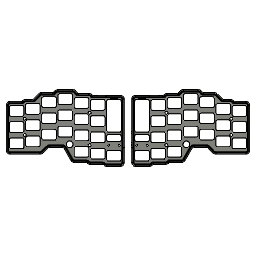
mriya-bumper-mjf-v1.17 (Autodesk Fusion 360 design; units mm, degrees)
Autodesk Fusion 360 part; units mm, degrees
(part 1 of 2)
sketch "mriya-bumper-mjf" plane through (0, 0, 0) normal (0, 0, 1) x (1, 0, 0)
  line L0 (-101.0213, 15.6719) -> (-94.7787, 21.9145) construction
  line L1 (-26.4858, 1.079) -> (-27.6142, 2.2074) construction
  line L2 (-138.1, 14.7932) -> (-103.1426, 14.7932) construction
  line L3 (-44.0716, 2.7932) -> (-29.0284, 2.7932) construction
  line L4 (-8.6, 0.4932) -> (-25.0716, 0.4932) construction
  line L5 (-64.4741, 6.1094) -> (-72.7517, 20.7608) construction
  line L6 (-45.4858, 3.379) -> (-46.6142, 4.5074) construction
  line L7 (-122.6142, 71.579) -> (-121.4858, 72.7074) construction
  line L8 (-101.0716, 81.2932) -> (-87.2284, 81.2932) construction
  line L9 (-138.1, 70.9932) -> (-124.0284, 70.9932) construction
  line L10 (-92.6574, 22.7932) -> (-76.2344, 22.7932) construction
  line L11 (-48.0284, 5.0932) -> (-62.7328, 5.0932) construction
  line L12 (-82.0716, 84.7932) -> (-64.7284, 84.7932) construction
  line L13 (-58.5716, 80.2932) -> (-45.7284, 80.2932) construction
  line L14 (-24.8, 19.4932) -> (-7.1, 19.4932) construction
  line L15 (-25.6, 20.2932) -> (-25.6, 77.9932) construction
  line L16 (-83.4858, 84.2074) -> (-85.8142, 81.879) construction
  line L17 (-63.3142, 84.2074) -> (-59.9858, 80.879) construction
  line L18 (-139.6, 69.4932) -> (-139.6, 16.2932) construction
  line L19 (-43.1858, 78.579) -> (-44.3142, 79.7074) construction
  line L20 (-99.4, 40.3932) -> (-99.4, 27.9932) construction
  line L21 (-98.6, 41.1932) -> (-86.2, 41.1932) construction
  line L22 (-98.6, 27.1932) -> (-86.2, 27.1932) construction
  line L23 (-85.4, 40.3932) -> (-85.4, 27.9932) construction
  line L24 (-42.4, 56.0932) -> (-42.4, 43.6932) construction
  line L25 (-41.6, 56.8932) -> (-29.2, 56.8932) construction
  line L26 (-41.6, 42.8932) -> (-29.2, 42.8932) construction
  line L27 (-28.4, 56.0932) -> (-28.4, 43.6932) construction
  line L28 (-61.4, 58.3932) -> (-61.4, 45.9932) construction
  line L29 (-60.6, 59.1932) -> (-48.2, 59.1932) construction
  line L30 (-60.6, 45.1932) -> (-48.2, 45.1932) construction
  line L31 (-47.4, 58.3932) -> (-47.4, 45.9932) construction
  line L32 (-137.4, 68.0932) -> (-137.4, 55.6932) construction
  line L33 (-136.6, 68.8932) -> (-124.2, 68.8932) construction
  line L34 (-136.6, 54.8932) -> (-124.2, 54.8932) construction
  line L35 (-123.4, 68.0932) -> (-123.4, 55.6932) construction
  line L36 (-61.4, 39.3932) -> (-61.4, 26.9932) construction
  line L37 (-60.6, 40.1932) -> (-48.2, 40.1932) construction
  line L38 (-60.6, 26.1932) -> (-48.2, 26.1932) construction
  line L39 (-47.4, 39.3932) -> (-47.4, 26.9932) construction
  line L40 (-42.4, 18.0932) -> (-42.4, 5.6932) construction
  line L41 (-41.6, 18.8932) -> (-29.2, 18.8932) construction
  line L42 (-41.6, 4.8932) -> (-29.2, 4.8932) construction
  line L43 (-28.4, 18.0932) -> (-28.4, 5.6932) construction
  line L44 (-23.4, 15.7932) -> (-23.4, 3.3932) construction
  line L45 (-22.6, 16.5932) -> (-10.2, 16.5932) construction
  line L46 (-22.6, 2.5932) -> (-10.2, 2.5932) construction
  line L47 (-9.4, 15.7932) -> (-9.4, 3.3932) construction
  line L48 (-137.4, 49.0932) -> (-137.4, 36.6932) construction
  line L49 (-136.6, 49.8932) -> (-124.2, 49.8932) construction
  line L50 (-136.6, 35.8932) -> (-124.2, 35.8932) construction
  line L51 (-123.4, 49.0932) -> (-123.4, 36.6932) construction
  line L52 (-118.4, 51.3932) -> (-118.4, 38.9932) construction
  line L53 (-117.6, 52.1932) -> (-105.2, 52.1932) construction
  line L54 (-117.6, 38.1932) -> (-105.2, 38.1932) construction
  line L55 (-104.4, 51.3932) -> (-104.4, 38.9932) construction
  line L56 (-137.4, 30.0932) -> (-137.4, 17.6932) construction
  line L57 (-136.6, 30.8932) -> (-124.2, 30.8932) construction
  line L58 (-136.6, 16.8932) -> (-124.2, 16.8932) construction
  line L59 (-123.4, 30.0932) -> (-123.4, 17.6932) construction
  line L60 (-61.4, 20.3932) -> (-61.4, 7.9932) construction
  line L61 (-60.6, 21.1932) -> (-48.2, 21.1932) construction
  line L62 (-60.6, 7.1932) -> (-48.2, 7.1932) construction
  line L63 (-47.4, 20.3932) -> (-47.4, 7.9932) construction
  line L64 (-80.4, 43.8932) -> (-80.4, 31.4932) construction
  line L65 (-79.6, 44.6932) -> (-67.2, 44.6932) construction
  line L66 (-79.6, 30.6932) -> (-67.2, 30.6932) construction
  line L67 (-66.4, 43.8932) -> (-66.4, 31.4932) construction
  line L68 (-80.4, 81.8932) -> (-80.4, 69.4932) construction
  line L69 (-79.6, 82.6932) -> (-67.2, 82.6932) construction
  line L70 (-79.6, 68.6932) -> (-67.2, 68.6932) construction
  line L71 (-66.4, 81.8932) -> (-66.4, 69.4932) construction
  line L72 (-42.4, 37.0932) -> (-42.4, 24.6932) construction
  line L73 (-41.6, 37.8932) -> (-29.2, 37.8932) construction
  line L74 (-41.6, 23.8932) -> (-29.2, 23.8932) construction
  line L75 (-28.4, 37.0932) -> (-28.4, 24.6932) construction
  line L76 (-118.4, 32.3932) -> (-118.4, 19.9932) construction
  line L77 (-117.6, 33.1932) -> (-105.2, 33.1932) construction
  line L78 (-117.6, 19.1932) -> (-105.2, 19.1932) construction
  line L79 (-104.4, 32.3932) -> (-104.4, 19.9932) construction
  line L80 (-61.4, 77.3932) -> (-61.4, 64.9932) construction
  line L81 (-60.6, 78.1932) -> (-48.2, 78.1932) construction
  line L82 (-60.6, 64.1932) -> (-48.2, 64.1932) construction
  line L83 (-47.4, 77.3932) -> (-47.4, 64.9932) construction
  line L84 (-42.4, 75.0932) -> (-42.4, 62.6932) construction
  line L85 (-41.6, 75.8932) -> (-29.2, 75.8932) construction
  line L86 (-41.6, 61.8932) -> (-29.2, 61.8932) construction
  line L87 (-28.4, 75.0932) -> (-28.4, 62.6932) construction
  line L88 (-118.4, 70.3932) -> (-118.4, 57.9932) construction
  line L89 (-117.6, 71.1932) -> (-105.2, 71.1932) construction
  line L90 (-117.6, 57.1932) -> (-105.2, 57.1932) construction
  line L91 (-104.4, 70.3932) -> (-104.4, 57.9932) construction
  line L92 (-99.4, 59.3932) -> (-99.4, 46.9932) construction
  line L93 (-98.6, 60.1932) -> (-86.2, 60.1932) construction
  line L94 (-98.6, 46.1932) -> (-86.2, 46.1932) construction
  line L95 (-85.4, 59.3932) -> (-85.4, 46.9932) construction
  line L96 (-80.4, 62.8932) -> (-80.4, 50.4932) construction
  line L97 (-79.6, 63.6932) -> (-67.2, 63.6932) construction
  line L98 (-79.6, 49.6932) -> (-67.2, 49.6932) construction
  line L99 (-66.4, 62.8932) -> (-66.4, 50.4932) construction
  line L100 (-99.4, 78.3932) -> (-99.4, 65.9932) construction
  line L101 (-98.6, 79.1932) -> (-86.2, 79.1932) construction
  line L102 (-98.6, 65.1932) -> (-86.2, 65.1932) construction
  line L103 (-85.4, 78.3932) -> (-85.4, 65.9932) construction
  circle A0 centre (-120.9, 53.5432) radius 1.7
  circle A1 centre (-120.9, 34.5432) radius 1.7
  circle A2 centre (-68.3, 23.4932) radius 3.9
  circle A3 centre (-44.9, 22.5432) radius 1.7
  circle A4 centre (-44.9, 60.5432) radius 1.7
  arc A5 (-43.1858, 78.579) -> (-41.7716, 77.9932) centre (-41.7716, 79.9932) ccw construction
  arc A6 (-44.3142, 79.7074) -> (-45.7284, 80.2932) centre (-45.7285, 78.2931) ccw construction
  arc A7 (-59.9858, 80.879) -> (-58.5716, 80.2932) centre (-58.5716, 82.2931) ccw construction
  arc A8 (-63.3142, 84.2074) -> (-64.7284, 84.7932) centre (-64.7285, 82.7931) ccw construction
  arc A9 (-82.0716, 84.7932) -> (-83.4858, 84.2074) centre (-82.0716, 82.7933) ccw construction
  arc A10 (-87.2284, 81.2932) -> (-85.8142, 81.879) centre (-87.2284, 83.2932) ccw construction
  arc A11 (-101.0716, 81.2932) -> (-102.4858, 80.7074) centre (-101.0716, 79.2933) ccw construction
  arc A12 (-120.0716, 73.2932) -> (-121.4858, 72.7074) centre (-120.0716, 71.2933) ccw construction
  arc A13 (-124.0284, 70.9932) -> (-122.6142, 71.579) centre (-124.0284, 72.9932) ccw construction
  arc A14 (-138.1, 70.9932) -> (-139.6, 69.4932) centre (-138.1, 69.4932) ccw construction
  arc A15 (-139.6, 16.2932) -> (-138.1, 14.7932) centre (-138.1, 16.2932) ccw construction
  arc A16 (-103.1426, 14.7932) -> (-101.0213, 15.6719) centre (-103.1426, 17.7931) ccw construction
  arc A17 (-92.6574, 22.7932) -> (-94.7787, 21.9145) centre (-92.6573, 19.7931) ccw construction
  arc A18 (-72.7517, 20.7608) -> (-76.2344, 22.7932) centre (-76.2344, 18.793) ccw construction
  arc A19 (-64.4741, 6.1094) -> (-62.7328, 5.0932) centre (-62.7328, 7.0932) ccw construction
  arc A20 (-46.6142, 4.5074) -> (-48.0284, 5.0932) centre (-48.0284, 3.0933) ccw construction
  arc A21 (-45.4858, 3.379) -> (-44.0716, 2.7932) centre (-44.0715, 4.7933) ccw construction
  arc A22 (-27.6142, 2.2074) -> (-29.0284, 2.7932) centre (-29.0284, 0.7933) ccw construction
  arc A23 (-26.4858, 1.079) -> (-25.0716, 0.4932) centre (-25.0715, 2.4933) ccw construction
  arc A24 (-8.6, 0.4932) -> (-7.1, 1.9932) centre (-8.6, 1.9932) ccw construction
  line L104 (-7.1, 1.9932) -> (-7.1, 76.4932) construction
  line L105 (-41.7716, 77.9932) -> (-8.6, 77.9932) construction
  arc A25 (-7.1, 76.4932) -> (-8.6, 77.9932) centre (-8.6, 76.4932) ccw construction
  arc A26 (-136.6, 68.8932) -> (-137.4, 68.0932) centre (-136.6, 68.0932) ccw construction
  arc A27 (-123.4, 68.0932) -> (-124.2, 68.8932) centre (-124.2, 68.0932) ccw construction
  arc A28 (-124.2, 54.8932) -> (-123.4, 55.6932) centre (-124.2, 55.6932) ccw construction
  arc A29 (-137.4, 55.6932) -> (-136.6, 54.8932) centre (-136.6, 55.6932) ccw construction
  arc A30 (-136.6, 49.8932) -> (-137.4, 49.0932) centre (-136.6, 49.0932) ccw construction
  arc A31 (-123.4, 49.0932) -> (-124.2, 49.8932) centre (-124.2, 49.0932) ccw construction
  arc A32 (-124.2, 35.8932) -> (-123.4, 36.6932) centre (-124.2, 36.6932) ccw construction
  arc A33 (-137.4, 36.6932) -> (-136.6, 35.8932) centre (-136.6, 36.6932) ccw construction
  arc A34 (-136.6, 30.8932) -> (-137.4, 30.0932) centre (-136.6, 30.0932) ccw construction
  arc A35 (-123.4, 30.0932) -> (-124.2, 30.8932) centre (-124.2, 30.0932) ccw construction
  arc A36 (-124.2, 16.8932) -> (-123.4, 17.6932) centre (-124.2, 17.6932) ccw construction
  arc A37 (-137.4, 17.6932) -> (-136.6, 16.8932) centre (-136.6, 17.6932) ccw construction
  arc A38 (-118.4, 19.9932) -> (-117.6, 19.1932) centre (-117.6, 19.9932) ccw construction
  arc A39 (-105.2, 19.1932) -> (-104.4, 19.9932) centre (-105.2, 19.9932) ccw construction
  arc A40 (-104.4, 32.3932) -> (-105.2, 33.1932) centre (-105.2, 32.3932) ccw construction
  arc A41 (-117.6, 33.1932) -> (-118.4, 32.3932) centre (-117.6, 32.3932) ccw construction
  arc A42 (-105.2, 38.1932) -> (-104.4, 38.9932) centre (-105.2, 38.9932) ccw construction
  arc A43 (-118.4, 38.9932) -> (-117.6, 38.1932) centre (-117.6, 38.9932) ccw construction
  arc A44 (-117.6, 52.1932) -> (-118.4, 51.3932) centre (-117.6, 51.3932) ccw construction
  arc A45 (-104.4, 51.3932) -> (-105.2, 52.1932) centre (-105.2, 51.3932) ccw construction
  arc A46 (-118.4, 57.9932) -> (-117.6, 57.1932) centre (-117.6, 57.9932) ccw construction
  arc A47 (-105.2, 57.1932) -> (-104.4, 57.9932) centre (-105.2, 57.9932) ccw construction
  arc A48 (-104.4, 70.3932) -> (-105.2, 71.1932) centre (-105.2, 70.3932) ccw construction
  arc A49 (-117.6, 71.1932) -> (-118.4, 70.3932) centre (-117.6, 70.3932) ccw construction
  arc A50 (-98.6, 79.1932) -> (-99.4, 78.3932) centre (-98.6, 78.3932) ccw construction
  arc A51 (-85.4, 78.3932) -> (-86.2, 79.1932) centre (-86.2, 78.3932) ccw construction
  arc A52 (-86.2, 65.1932) -> (-85.4, 65.9932) centre (-86.2, 65.9932) ccw construction
  arc A53 (-99.4, 65.9932) -> (-98.6, 65.1932) centre (-98.6, 65.9932) ccw construction
  arc A54 (-98.6, 60.1932) -> (-99.4, 59.3932) centre (-98.6, 59.3932) ccw construction
  arc A55 (-85.4, 59.3932) -> (-86.2, 60.1932) centre (-86.2, 59.3932) ccw construction
  arc A56 (-86.2, 46.1932) -> (-85.4, 46.9932) centre (-86.2, 46.9932) ccw construction
  arc A57 (-99.4, 46.9932) -> (-98.6, 46.1932) centre (-98.6, 46.9932) ccw construction
  arc A58 (-98.6, 41.1932) -> (-99.4, 40.3932) centre (-98.6, 40.3932) ccw construction
  arc A59 (-99.4, 27.9932) -> (-98.6, 27.1932) centre (-98.6, 27.9932) ccw construction
  arc A60 (-86.2, 27.1932) -> (-85.4, 27.9932) centre (-86.2, 27.9932) ccw construction
  arc A61 (-85.4, 40.3932) -> (-86.2, 41.1932) centre (-86.2, 40.3932) ccw construction
  arc A62 (-80.4, 31.4932) -> (-79.6, 30.6932) centre (-79.6, 31.4932) ccw construction
  arc A63 (-79.6, 44.6932) -> (-80.4, 43.8932) centre (-79.6, 43.8932) ccw construction
  arc A64 (-66.4, 43.8932) -> (-67.2, 44.6932) centre (-67.2, 43.8932) ccw construction
  arc A65 (-67.2, 30.6932) -> (-66.4, 31.4932) centre (-67.2, 31.4932) ccw construction
  arc A66 (-67.2, 49.6932) -> (-66.4, 50.4932) centre (-67.2, 50.4932) ccw construction
  arc A67 (-80.4, 50.4932) -> (-79.6, 49.6932) centre (-79.6, 50.4932) ccw construction
  arc A68 (-79.6, 63.6932) -> (-80.4, 62.8932) centre (-79.6, 62.8932) ccw construction
  arc A69 (-66.4, 62.8932) -> (-67.2, 63.6932) centre (-67.2, 62.8932) ccw construction
  arc A70 (-67.2, 68.6932) -> (-66.4, 69.4932) centre (-67.2, 69.4932) ccw construction
  arc A71 (-80.4, 69.4932) -> (-79.6, 68.6932) centre (-79.6, 69.4932) ccw construction
  arc A72 (-79.6, 82.6932) -> (-80.4, 81.8932) centre (-79.6, 81.8932) ccw construction
  arc A73 (-66.4, 81.8932) -> (-67.2, 82.6932) centre (-67.2, 81.8932) ccw construction
  arc A74 (-60.6, 78.1932) -> (-61.4, 77.3932) centre (-60.6, 77.3932) ccw construction
  arc A75 (-61.4, 64.9932) -> (-60.6, 64.1932) centre (-60.6, 64.9932) ccw construction
  arc A76 (-48.2, 64.1932) -> (-47.4, 64.9932) centre (-48.2, 64.9932) ccw construction
  arc A77 (-47.4, 77.3932) -> (-48.2, 78.1932) centre (-48.2, 77.3932) ccw construction
  arc A78 (-47.4, 58.3932) -> (-48.2, 59.1932) centre (-48.2, 58.3932) ccw construction
  arc A79 (-60.6, 59.1932) -> (-61.4, 58.3932) centre (-60.6, 58.3932) ccw construction
  arc A80 (-61.4, 45.9932) -> (-60.6, 45.1932) centre (-60.6, 45.9932) ccw construction
  arc A81 (-48.2, 45.1932) -> (-47.4, 45.9932) centre (-48.2, 45.9932) ccw construction
  arc A82 (-47.4, 39.3932) -> (-48.2, 40.1932) centre (-48.2, 39.3932) ccw construction
  arc A83 (-60.6, 40.1932) -> (-61.4, 39.3932) centre (-60.6, 39.3932) ccw construction
  arc A84 (-61.4, 26.9932) -> (-60.6, 26.1932) centre (-60.6, 26.9932) ccw construction
  arc A85 (-48.2, 26.1932) -> (-47.4, 26.9932) centre (-48.2, 26.9932) ccw construction
  arc A86 (-47.4, 20.3932) -> (-48.2, 21.1932) centre (-48.2, 20.3932) ccw construction
  arc A87 (-60.6, 21.1932) -> (-61.4, 20.3932) centre (-60.6, 20.3932) ccw construction
  arc A88 (-61.4, 7.9932) -> (-60.6, 7.1932) centre (-60.6, 7.9932) ccw construction
  arc A89 (-48.2, 7.1932) -> (-47.4, 7.9932) centre (-48.2, 7.9932) ccw construction
  arc A90 (-42.4, 5.6932) -> (-41.6, 4.8932) centre (-41.6, 5.6932) ccw construction
  arc A91 (-29.2, 4.8932) -> (-28.4, 5.6932) centre (-29.2, 5.6932) ccw construction
  arc A92 (-28.4, 18.0932) -> (-29.2, 18.8932) centre (-29.2, 18.0932) ccw construction
  arc A93 (-41.6, 18.8932) -> (-42.4, 18.0932) centre (-41.6, 18.0932) ccw construction
  arc A94 (-23.4, 3.3932) -> (-22.6, 2.5932) centre (-22.6, 3.3932) ccw construction
  arc A95 (-10.2, 2.5932) -> (-9.4, 3.3932) centre (-10.2, 3.3932) ccw construction
  arc A96 (-9.4, 15.7932) -> (-10.2, 16.5932) centre (-10.2, 15.7932) ccw construction
  arc A97 (-22.6, 16.5932) -> (-23.4, 15.7932) centre (-22.6, 15.7932) ccw construction
  arc A98 (-29.2, 23.8932) -> (-28.4, 24.6932) centre (-29.2, 24.6932) ccw construction
  arc A99 (-42.4, 24.6932) -> (-41.6, 23.8932) centre (-41.6, 24.6932) ccw construction
  arc A100 (-41.6, 37.8932) -> (-42.4, 37.0932) centre (-41.6, 37.0932) ccw construction
  arc A101 (-28.4, 37.0932) -> (-29.2, 37.8932) centre (-29.2, 37.0932) ccw construction
  arc A102 (-29.2, 42.8932) -> (-28.4, 43.6932) centre (-29.2, 43.6932) ccw construction
  arc A103 (-42.4, 43.6932) -> (-41.6, 42.8932) centre (-41.6, 43.6932) ccw construction
  arc A104 (-41.6, 56.8932) -> (-42.4, 56.0932) centre (-41.6, 56.0932) ccw construction
  arc A105 (-28.4, 56.0932) -> (-29.2, 56.8932) centre (-29.2, 56.0932) ccw construction
  arc A106 (-29.2, 61.8932) -> (-28.4, 62.6932) centre (-29.2, 62.6932) ccw construction
  arc A107 (-42.4, 62.6932) -> (-41.6, 61.8932) centre (-41.6, 62.6932) ccw construction
  arc A108 (-41.6, 75.8932) -> (-42.4, 75.0932) centre (-41.6, 75.0932) ccw construction
  arc A109 (-28.4, 75.0932) -> (-29.2, 75.8932) centre (-29.2, 75.0932) ccw construction
  circle A110 centre (-22.6, 22.4932) radius 1.1
  circle A111 centre (-10.1, 22.4932) radius 1.1
  line L106 (-102.4858, 80.7074) -> (-109.0213, 74.1719) construction
  line L107 (-120.0716, 73.2932) -> (-111.1426, 73.2932) construction
  arc A112 (-111.1426, 73.2932) -> (-109.0213, 74.1719) centre (-111.1426, 76.2932) ccw construction
  arc A113 (-64.7284, 82.7932) -> (-64.7285, 82.7932) centre (-64.7285, 82.7931) ccw
  arc A114 (-45.7284, 78.2932) -> (-45.7285, 78.2932) centre (-45.7285, 78.2931) ccw
  arc A115 (-25.0716, 2.4932) -> (-25.0715, 2.4932) centre (-25.0715, 2.4933) ccw
  arc A116 (-44.0716, 4.7932) -> (-44.0715, 4.7932) centre (-44.0715, 4.7933) ccw
  line L108 (-138.9, 58.3932) -> (-138.9, 66.8932)
  line L109 (-136.9, 68.8932) -> (-123.9, 68.8932)
  arc A117 (-121.9, 66.8932) -> (-123.9, 68.8932) centre (-123.9, 66.8932) ccw
  arc A118 (-136.9, 68.8932) -> (-138.9, 66.8932) centre (-136.9, 66.8932) ccw
  line L110 (-104.9, 58.6932) -> (-117.9, 58.6932)
  line L111 (-119.9, 60.6932) -> (-119.9, 69.1932)
  arc A119 (-117.9, 71.1932) -> (-119.9, 69.1932) centre (-117.9, 69.1932) ccw
  line L112 (-117.9, 71.1932) -> (-104.9, 71.1932)
  arc A120 (-102.9, 69.1932) -> (-104.9, 71.1932) centre (-104.9, 69.1932) ccw
  line L113 (-102.9, 69.1932) -> (-102.9, 60.6932)
  line L114 (-85.9, 66.6932) -> (-98.9, 66.6932)
  line L115 (-100.9, 68.6932) -> (-100.9, 77.1932)
  arc A121 (-98.9, 79.1932) -> (-100.9, 77.1932) centre (-98.9, 77.1932) ccw
  line L116 (-98.9, 79.1932) -> (-85.9, 79.1932)
  arc A122 (-83.9, 77.1932) -> (-85.9, 79.1932) centre (-85.9, 77.1932) ccw
  line L117 (-83.9, 77.1932) -> (-83.9, 68.6932)
  line L118 (-66.9, 70.1932) -> (-79.9, 70.1932)
  line L119 (-81.9, 72.1932) -> (-81.9, 80.6932)
  arc A123 (-79.9, 82.6932) -> (-81.9, 80.6932) centre (-79.9, 80.6932) ccw
  line L120 (-79.9, 82.6932) -> (-66.9, 82.6932)
  arc A124 (-64.9, 80.6932) -> (-66.9, 82.6932) centre (-66.9, 80.6932) ccw
  line L121 (-64.9, 80.6932) -> (-64.9, 72.1932)
  line L122 (-47.9, 65.6932) -> (-60.9, 65.6932)
  line L123 (-62.9, 67.6932) -> (-62.9, 76.1932)
  arc A125 (-60.9, 78.1932) -> (-62.9, 76.1932) centre (-60.9, 76.1932) ccw
  line L124 (-60.9, 78.1932) -> (-47.9, 78.1932)
  arc A126 (-45.9, 76.1932) -> (-47.9, 78.1932) centre (-47.9, 76.1932) ccw
  line L125 (-45.9, 76.1932) -> (-45.9, 67.6932)
  line L126 (-43.9, 65.3932) -> (-43.9, 73.8932)
  arc A127 (-41.9, 75.8932) -> (-43.9, 73.8932) centre (-41.9, 73.8932) ccw
  line L127 (-41.9, 75.8932) -> (-28.9, 75.8932)
  arc A128 (-26.9, 73.8932) -> (-28.9, 75.8932) centre (-28.9, 73.8932) ccw
  line L128 (-26.9, 73.8932) -> (-26.9, 65.3932)
  arc A129 (-9.9, 26.8932) -> (-7.9, 28.8932) centre (-9.9, 28.8932) ccw
  line L129 (-9.9, 26.8932) -> (-22.9, 26.8932)
  arc A130 (-24.9, 28.8932) -> (-22.9, 26.8932) centre (-22.9, 28.8932) ccw
  arc A131 (-22.9, 75.8932) -> (-24.9, 73.8932) centre (-22.9, 73.8932) ccw
  arc A132 (-7.9, 73.8932) -> (-9.9, 75.8932) centre (-9.9, 73.8932) ccw
  line L130 (-28.9, 63.3932) -> (-41.9, 63.3932)
  line L131 (-121.9, 66.8932) -> (-121.9, 58.3932)
  line L132 (-123.9, 56.3932) -> (-136.9, 56.3932)
  line L133 (-122.6849, 71.6497) -> (-121.5565, 72.7781)
  arc A133 (-120.0716, 73.3932) -> (-121.5565, 72.7781) centre (-120.0716, 71.2933) ccw
  line L134 (-120.0716, 73.3932) -> (-111.1426, 73.3932)
  arc A134 (-111.1426, 73.3932) -> (-109.092, 74.2426) centre (-111.1426, 76.2932) ccw
  line L135 (-102.5565, 80.7781) -> (-109.092, 74.2426)
  arc A135 (-101.0716, 81.3932) -> (-102.5565, 80.7781) centre (-101.0716, 79.2933) ccw
  line L136 (-101.0716, 81.3932) -> (-87.2284, 81.3932)
  arc A136 (-87.2284, 81.3932) -> (-85.8849, 81.9497) centre (-87.2284, 83.2932) ccw
  line L137 (-83.5565, 84.2781) -> (-85.8849, 81.9497)
  arc A137 (-82.0716, 84.8932) -> (-83.5565, 84.2781) centre (-82.0716, 82.7933) ccw
  line L138 (-82.0716, 84.8932) -> (-64.7284, 84.8932)
  arc A138 (-63.2435, 84.2781) -> (-64.7284, 84.8932) centre (-64.7285, 82.7931) ccw
  line L139 (-63.2435, 84.2781) -> (-59.9151, 80.9497)
  arc A139 (-59.9151, 80.9497) -> (-58.5716, 80.3932) centre (-58.5716, 82.2931) ccw
  line L140 (-58.5716, 80.3932) -> (-45.7284, 80.3932)
  arc A140 (-44.2435, 79.7781) -> (-45.7284, 80.3932) centre (-45.7285, 78.2931) ccw
  line L141 (-43.1151, 78.6497) -> (-44.2435, 79.7781)
  arc A141 (-43.1151, 78.6497) -> (-41.7716, 78.0932) centre (-41.7716, 79.9932) ccw
  line L142 (-41.7716, 78.0932) -> (-8.6, 78.0932)
  arc A142 (-7, 76.4932) -> (-8.6, 78.0932) centre (-8.6, 76.4932) ccw
  line L143 (-7, 1.9932) -> (-7, 76.4932)
  arc A143 (-8.6, 0.3932) -> (-7, 1.9932) centre (-8.6, 1.9932) ccw
  line L144 (-8.6, 0.3932) -> (-25.0716, 0.3932)
  arc A144 (-26.5565, 1.0083) -> (-25.0716, 0.3932) centre (-25.0715, 2.4933) ccw
  line L145 (-26.5565, 1.0083) -> (-27.6849, 2.1367)
  arc A145 (-27.6849, 2.1367) -> (-29.0284, 2.6932) centre (-29.0284, 0.7933) ccw
  line L146 (-44.0716, 2.6932) -> (-29.0284, 2.6932)
  arc A146 (-45.5565, 3.3083) -> (-44.0716, 2.6932) centre (-44.0715, 4.7933) ccw
  line L147 (-45.5565, 3.3083) -> (-46.6849, 4.4367)
  arc A147 (-46.6849, 4.4367) -> (-48.0284, 4.9932) centre (-48.0284, 3.0933) ccw
  line L148 (-48.0284, 4.9932) -> (-62.7328, 4.9932)
  arc A148 (-64.5612, 6.0602) -> (-62.7328, 4.9932) centre (-62.7328, 7.0932) ccw
  line L149 (-64.5612, 6.0602) -> (-72.8388, 20.7116)
  arc A149 (-72.8388, 20.7116) -> (-76.2344, 22.6932) centre (-76.2344, 18.793) ccw
  line L150 (-92.6574, 22.6932) -> (-76.2344, 22.6932)
  arc A150 (-92.6574, 22.6932) -> (-94.708, 21.8438) centre (-92.6573, 19.7931) ccw
  line L151 (-100.9506, 15.6012) -> (-94.708, 21.8438)
  arc A151 (-103.1426, 14.6932) -> (-100.9506, 15.6012) centre (-103.1426, 17.7931) ccw
  line L152 (-138.1, 14.6932) -> (-103.1426, 14.6932)
  arc A152 (-139.7, 16.2932) -> (-138.1, 14.6932) centre (-138.1, 16.2932) ccw
  line L153 (-139.7, 69.4932) -> (-139.7, 16.2932)
  arc A153 (-138.1, 71.0932) -> (-139.7, 69.4932) centre (-138.1, 69.4932) ccw
  line L154 (-138.1, 71.0932) -> (-124.0284, 71.0932)
  arc A154 (-124.0284, 71.0932) -> (-122.6849, 71.6497) centre (-124.0284, 72.9932) ccw
  line L155 (-22.9, 34.8932) -> (-9.9, 34.8932)
  line L156 (-24.9, 28.8932) -> (-24.9, 32.8932)
  line L157 (-24.9, 39.8932) -> (-24.9, 73.8932)
  line L158 (-7.9, 73.8932) -> (-7.9, 39.8932)
  line L159 (-7.9, 32.8932) -> (-7.9, 28.8932)
  arc A155 (-24.9, 39.8932) -> (-22.9, 37.8932) centre (-22.9, 39.8932) ccw
  arc A156 (-9.9, 37.8932) -> (-7.9, 39.8932) centre (-9.9, 39.8932) ccw
  arc A157 (-22.9, 34.8932) -> (-24.9, 32.8932) centre (-22.9, 32.8932) ccw
  arc A158 (-7.9, 32.8932) -> (-9.9, 34.8932) centre (-9.9, 32.8932) ccw
  circle A159 centre (-22.6, 22.4932) radius 2.1
  circle A160 centre (-10.1, 22.4932) radius 2.1
  arc A161 (-25.6, 20.2932) -> (-24.8, 19.4932) centre (-24.8, 20.2932) ccw construction
  arc A162 (-138.9, 58.3932) -> (-136.9, 56.3932) centre (-136.9, 58.3932) ccw
  arc A163 (-123.9, 56.3932) -> (-121.9, 58.3932) centre (-123.9, 58.3932) ccw
  arc A164 (-119.9, 60.6932) -> (-117.9, 58.6932) centre (-117.9, 60.6932) ccw
  arc A165 (-104.9, 58.6932) -> (-102.9, 60.6932) centre (-104.9, 60.6932) ccw
  arc A166 (-100.9, 68.6932) -> (-98.9, 66.6932) centre (-98.9, 68.6932) ccw
  arc A167 (-85.9, 66.6932) -> (-83.9, 68.6932) centre (-85.9, 68.6932) ccw
  arc A168 (-81.9, 72.1932) -> (-79.9, 70.1932) centre (-79.9, 72.1932) ccw
  arc A169 (-66.9, 70.1932) -> (-64.9, 72.1932) centre (-66.9, 72.1932) ccw
  arc A170 (-62.9, 67.6932) -> (-60.9, 65.6932) centre (-60.9, 67.6932) ccw
  arc A171 (-47.9, 65.6932) -> (-45.9, 67.6932) centre (-47.9, 67.6932) ccw
  arc A172 (-43.9, 65.3932) -> (-41.9, 63.3932) centre (-41.9, 65.3932) ccw
  arc A173 (-28.9, 63.3932) -> (-26.9, 65.3932) centre (-28.9, 65.3932) ccw
  line L160 (-121.9, 47.8932) -> (-121.9, 39.3932)
  arc A174 (-121.9, 47.8932) -> (-123.9, 49.8932) centre (-123.9, 47.8932) ccw
  line L161 (-136.9, 49.8932) -> (-123.9, 49.8932)
  arc A175 (-136.9, 49.8932) -> (-138.9, 47.8932) centre (-136.9, 47.8932) ccw
  line L162 (-138.9, 39.3932) -> (-138.9, 47.8932)
  arc A176 (-138.9, 39.3932) -> (-136.9, 37.3932) centre (-136.9, 39.3932) ccw
  line L163 (-123.9, 37.3932) -> (-136.9, 37.3932)
  arc A177 (-123.9, 37.3932) -> (-121.9, 39.3932) centre (-123.9, 39.3932) ccw
  arc A178 (-104.9, 39.6932) -> (-102.9, 41.6932) centre (-104.9, 41.6932) ccw
  line L164 (-104.9, 39.6932) -> (-117.9, 39.6932)
  arc A179 (-119.9, 41.6932) -> (-117.9, 39.6932) centre (-117.9, 41.6932) ccw
  line L165 (-119.9, 41.6932) -> (-119.9, 49.7719)
  line L166 (-117.4787, 52.1932) -> (-104.9, 52.1932)
  arc A180 (-102.9, 50.1932) -> (-104.9, 52.1932) centre (-104.9, 50.1932) ccw
  line L167 (-102.9, 50.1932) -> (-102.9, 41.6932)
  arc A181 (-85.9, 47.6932) -> (-83.9, 49.6932) centre (-85.9, 49.6932) ccw
  line L168 (-85.9, 47.6932) -> (-98.9, 47.6932)
  arc A182 (-100.9, 49.6932) -> (-98.9, 47.6932) centre (-98.9, 49.6932) ccw
  line L169 (-100.9, 49.6932) -> (-100.9, 58.1932)
  arc A183 (-98.9, 60.1932) -> (-100.9, 58.1932) centre (-98.9, 58.1932) ccw
  line L170 (-98.9, 60.1932) -> (-85.9, 60.1932)
  arc A184 (-83.9, 58.1932) -> (-85.9, 60.1932) centre (-85.9, 58.1932) ccw
  line L171 (-83.9, 58.1932) -> (-83.9, 49.6932)
  arc A185 (-79.9, 63.6932) -> (-81.9, 61.6932) centre (-79.9, 61.6932) ccw
  line L172 (-79.9, 63.6932) -> (-66.9, 63.6932)
  arc A186 (-64.9, 61.6932) -> (-66.9, 63.6932) centre (-66.9, 61.6932) ccw
  line L173 (-64.9, 61.6932) -> (-64.9, 53.1932)
  arc A187 (-66.9, 51.1932) -> (-64.9, 53.1932) centre (-66.9, 53.1932) ccw
  line L174 (-66.9, 51.1932) -> (-79.9, 51.1932)
  arc A188 (-81.9, 53.1932) -> (-79.9, 51.1932) centre (-79.9, 53.1932) ccw
  line L175 (-81.9, 53.1932) -> (-81.9, 61.6932)
  arc A189 (-60.9, 59.1932) -> (-62.9, 57.1932) centre (-60.9, 57.1932) ccw
  line L176 (-60.9, 59.1932) -> (-48.3213, 59.1932)
  line L177 (-45.9, 56.7719) -> (-45.9, 48.6932)
  arc A190 (-47.9, 46.6932) -> (-45.9, 48.6932) centre (-47.9, 48.6932) ccw
  line L178 (-47.9, 46.6932) -> (-60.9, 46.6932)
  arc A191 (-62.9, 48.6932) -> (-60.9, 46.6932) centre (-60.9, 48.6932) ccw
  line L179 (-62.9, 48.6932) -> (-62.9, 57.1932)
  arc A192 (-41.9, 56.8932) -> (-43.9, 54.8932) centre (-41.9, 54.8932) ccw
  line L180 (-41.9, 56.8932) -> (-28.9, 56.8932)
  arc A193 (-26.9, 54.8932) -> (-28.9, 56.8932) centre (-28.9, 54.8932) ccw
  line L181 (-26.9, 54.8932) -> (-26.9, 46.3932)
  arc A194 (-28.9, 44.3932) -> (-26.9, 46.3932) centre (-28.9, 46.3932) ccw
  line L182 (-28.9, 44.3932) -> (-41.9, 44.3932)
  arc A195 (-43.9, 46.3932) -> (-41.9, 44.3932) centre (-41.9, 46.3932) ccw
  line L183 (-43.9, 46.3932) -> (-43.9, 54.8932)
  arc A196 (-123.9, 18.3932) -> (-121.9, 20.3932) centre (-123.9, 20.3932) ccw
  line L184 (-123.9, 18.3932) -> (-136.9, 18.3932)
  arc A197 (-138.9, 20.3932) -> (-136.9, 18.3932) centre (-136.9, 20.3932) ccw
  line L185 (-138.9, 20.3932) -> (-138.9, 28.8932)
  arc A198 (-136.9, 30.8932) -> (-138.9, 28.8932) centre (-136.9, 28.8932) ccw
  line L186 (-136.9, 30.8932) -> (-123.9, 30.8932)
  arc A199 (-121.9, 28.8932) -> (-123.9, 30.8932) centre (-123.9, 28.8932) ccw
  line L187 (-121.9, 28.8932) -> (-121.9, 20.3932)
  arc A200 (-104.9, 20.6932) -> (-102.9, 22.6932) centre (-104.9, 22.6932) ccw
  line L188 (-104.9, 20.6932) -> (-117.9, 20.6932)
  arc A201 (-119.9, 22.6932) -> (-117.9, 20.6932) centre (-117.9, 22.6932) ccw
  line L189 (-119.9, 22.6932) -> (-119.9, 30.7719)
  line L190 (-117.4787, 33.1932) -> (-104.9, 33.1932)
  arc A202 (-102.9, 31.1932) -> (-104.9, 33.1932) centre (-104.9, 31.1932) ccw
  line L191 (-102.9, 31.1932) -> (-102.9, 22.6932)
  arc A203 (-85.9, 28.6932) -> (-83.9, 30.6932) centre (-85.9, 30.6932) ccw
  line L192 (-85.9, 28.6932) -> (-98.9, 28.6932)
  arc A204 (-100.9, 30.6932) -> (-98.9, 28.6932) centre (-98.9, 30.6932) ccw
  line L193 (-100.9, 30.6932) -> (-100.9, 39.1932)
  arc A205 (-98.9, 41.1932) -> (-100.9, 39.1932) centre (-98.9, 39.1932) ccw
  line L194 (-98.9, 41.1932) -> (-85.9, 41.1932)
  arc A206 (-83.9, 39.1932) -> (-85.9, 41.1932) centre (-85.9, 39.1932) ccw
  line L195 (-83.9, 39.1932) -> (-83.9, 30.6932)
  arc A207 (-66.9, 32.1932) -> (-64.9, 34.1932) centre (-66.9, 34.1932) ccw
  line L196 (-66.9, 32.1932) -> (-79.9, 32.1932)
  arc A208 (-81.9, 34.1932) -> (-79.9, 32.1932) centre (-79.9, 34.1932) ccw
  line L197 (-81.9, 34.1932) -> (-81.9, 42.6932)
  arc A209 (-79.9, 44.6932) -> (-81.9, 42.6932) centre (-79.9, 42.6932) ccw
  line L198 (-79.9, 44.6932) -> (-66.9, 44.6932)
  arc A210 (-64.9, 42.6932) -> (-66.9, 44.6932) centre (-66.9, 42.6932) ccw
  line L199 (-64.9, 42.6932) -> (-64.9, 34.1932)
  arc A211 (-47.9, 27.6932) -> (-45.9, 29.6932) centre (-47.9, 29.6932) ccw
  line L200 (-47.9, 27.6932) -> (-60.9, 27.6932)
  arc A212 (-62.9, 29.6932) -> (-60.9, 27.6932) centre (-60.9, 29.6932) ccw
  line L201 (-62.9, 29.6932) -> (-62.9, 38.1932)
  arc A213 (-60.9, 40.1932) -> (-62.9, 38.1932) centre (-60.9, 38.1932) ccw
  line L202 (-60.9, 40.1932) -> (-47.9, 40.1932)
  arc A214 (-45.9, 38.1932) -> (-47.9, 40.1932) centre (-47.9, 38.1932) ccw
  line L203 (-45.9, 38.1932) -> (-45.9, 29.6932)
  arc A215 (-28.9, 25.3932) -> (-26.9, 27.3932) centre (-28.9, 27.3932) ccw
  line L204 (-28.9, 25.3932) -> (-41.9, 25.3932)
  arc A216 (-43.9, 27.3932) -> (-41.9, 25.3932) centre (-41.9, 27.3932) ccw
  line L205 (-43.9, 27.3932) -> (-43.9, 35.8932)
  arc A217 (-41.9, 37.8932) -> (-43.9, 35.8932) centre (-41.9, 35.8932) ccw
  line L206 (-41.9, 37.8932) -> (-28.9, 37.8932)
  arc A218 (-26.9, 35.8932) -> (-28.9, 37.8932) centre (-28.9, 35.8932) ccw
  line L207 (-26.9, 35.8932) -> (-26.9, 27.3932)
  arc A219 (-60.9, 21.1932) -> (-62.9, 19.1932) centre (-60.9, 19.1932) ccw
  line L208 (-62.9, 10.6932) -> (-62.9, 19.1932)
  arc A220 (-62.9, 10.6932) -> (-60.9, 8.6932) centre (-60.9, 10.6932) ccw
  line L209 (-47.9, 8.6932) -> (-60.9, 8.6932)
  arc A221 (-47.9, 8.6932) -> (-45.9, 10.6932) centre (-47.9, 10.6932) ccw
  line L210 (-28.9, 6.3932) -> (-41.9, 6.3932)
  arc A222 (-28.9, 6.3932) -> (-26.9, 8.3932) centre (-28.9, 8.3932) ccw
  line L211 (-26.9, 16.8932) -> (-26.9, 8.3932)
  arc A223 (-26.9, 16.8932) -> (-28.9, 18.8932) centre (-28.9, 16.8932) ccw
  line L212 (-41.9, 18.8932) -> (-28.9, 18.8932)
  arc A224 (-41.9, 18.8932) -> (-43.9, 16.8932) centre (-41.9, 16.8932) ccw
  line L213 (-43.9, 8.3932) -> (-43.9, 16.8932)
  arc A225 (-43.9, 8.3932) -> (-41.9, 6.3932) centre (-41.9, 8.3932) ccw
  arc A226 (-9.9, 4.0932) -> (-7.9, 6.0932) centre (-9.9, 6.0932) ccw
  line L214 (-9.9, 4.0932) -> (-22.9, 4.0932)
  arc A227 (-24.9, 6.0932) -> (-22.9, 4.0932) centre (-22.9, 6.0932) ccw
  line L215 (-24.9, 6.0932) -> (-24.9, 14.5932)
  arc A228 (-22.9, 16.5932) -> (-24.9, 14.5932) centre (-22.9, 14.5932) ccw
  line L216 (-22.9, 16.5932) -> (-9.9, 16.5932)
  arc A229 (-7.9, 14.5932) -> (-9.9, 16.5932) centre (-9.9, 14.5932) ccw
  line L217 (-7.9, 14.5932) -> (-7.9, 6.0932)
  line L218 (-60.9, 21.1932) -> (-48.3213, 21.1932)
  line L219 (-45.9, 18.7719) -> (-45.9, 10.6932)
  line L220 (-47.2607, 20.7539) -> (-46.3393, 19.8325)
  arc A230 (-47.2607, 20.7539) -> (-48.3213, 21.1932) centre (-48.3213, 19.6932) ccw
  arc A231 (-45.9, 18.7719) -> (-46.3393, 19.8325) centre (-47.4, 18.7719) ccw
  line L221 (-47.2607, 58.7539) -> (-46.3393, 57.8325)
  arc A232 (-47.2607, 58.7539) -> (-48.3213, 59.1932) centre (-48.3213, 57.6932) ccw
  arc A233 (-45.9, 56.7719) -> (-46.3393, 57.8325) centre (-47.4, 56.7719) ccw
  line L222 (-119.4607, 31.8325) -> (-118.5393, 32.7539)
  arc A234 (-119.4607, 31.8325) -> (-119.9, 30.7719) centre (-118.4, 30.7719) ccw
  arc A235 (-117.4787, 33.1932) -> (-118.5393, 32.7539) centre (-117.4787, 31.6932) ccw
  line L223 (-119.4607, 50.8325) -> (-118.5393, 51.7539)
  arc A236 (-117.4787, 52.1932) -> (-118.5393, 51.7539) centre (-117.4787, 50.6932) ccw
  arc A237 (-119.4607, 50.8325) -> (-119.9, 49.7719) centre (-118.4, 49.7719) ccw
  line L224 (-22.9, 75.8932) -> (-9.9, 75.8932)
  line L225 (-22.9, 37.8932) -> (-9.9, 37.8932)
  arc A238 (-101.0716, 83.9932) -> (-104.395, 82.6166) centre (-101.0716, 79.2933) ccw
  line L226 (-101.0716, 83.9932) -> (-88.1397, 83.9932)
  line L227 (-85.395, 86.1166) -> (-87.079, 84.4325)
  arc A239 (-82.0716, 87.4932) -> (-85.395, 86.1166) centre (-82.0716, 82.7933) ccw
  line L228 (-82.0716, 87.4932) -> (-64.7284, 87.4932)
  arc A240 (-61.405, 86.1166) -> (-64.7284, 87.4932) centre (-64.7285, 82.7931) ccw
  line L229 (-61.405, 86.1166) -> (-58.721, 83.4325)
  line L230 (-57.6603, 82.9932) -> (-45.7284, 82.9932)
  arc A241 (-42.405, 81.6166) -> (-45.7284, 82.9932) centre (-45.7285, 78.2931) ccw
  line L231 (-41.921, 81.1325) -> (-42.405, 81.6166)
  line L232 (-40.8603, 80.6932) -> (-8.6, 80.6932)
  arc A242 (-4.4, 76.4932) -> (-8.6, 80.6932) centre (-8.6, 76.4932) ccw
  line L233 (-4.4, 1.9932) -> (-4.4, 76.4932)
  arc A243 (-8.6, -2.2068) -> (-4.4, 1.9932) centre (-8.6, 1.9932) ccw
  line L234 (-8.6, -2.2068) -> (-25.0716, -2.2068)
  arc A244 (-28.395, -0.8302) -> (-25.0716, -2.2068) centre (-25.0715, 2.4933) ccw
  line L235 (-28.395, -0.8302) -> (-28.879, -0.3461)
  line L236 (-44.0716, 0.0932) -> (-29.9397, 0.0932)
  arc A245 (-47.395, 1.4698) -> (-44.0716, 0.0932) centre (-44.0715, 4.7933) ccw
  line L237 (-47.395, 1.4698) -> (-47.879, 1.9539)
  line L238 (-48.9397, 2.3932) -> (-62.7328, 2.3932)
  arc A246 (-66.8249, 4.7813) -> (-62.7328, 2.3932) centre (-62.7328, 7.0932) ccw
  arc A247 (-103.1426, 12.0932) -> (-99.1121, 13.7627) centre (-103.1426, 17.7931) ccw
  line L239 (-138.1, 12.0932) -> (-103.1426, 12.0932)
  arc A248 (-142.3, 16.2932) -> (-138.1, 12.0932) centre (-138.1, 16.2932) ccw
  line L240 (-142.3, 69.4932) -> (-142.3, 16.2932)
  arc A249 (-138.1, 73.6932) -> (-142.3, 69.4932) centre (-138.1, 69.4932) ccw
  line L241 (-138.1, 73.6932) -> (-124.9397, 73.6932)
  line L242 (-123.879, 74.1325) -> (-123.395, 74.6166)
  arc A250 (-120.0716, 75.9932) -> (-123.395, 74.6166) centre (-120.0716, 71.2933) ccw
  line L243 (-99.1121, 13.7627) -> (-93.3674, 19.5074)
  line L244 (-91.9532, 20.0932) -> (-77.2264, 20.0932)
  line L245 (-66.8249, 4.7813) -> (-74.6144, 18.5689)
  line L246 (-20.7, 77.3932) -> (-12.1, 77.3932)
  arc A251 (-21.4, 78.0932) -> (-20.7, 77.3932) centre (-20.7, 78.0932) ccw
  arc A252 (-12.1, 77.3932) -> (-11.4, 78.0932) centre (-12.1, 78.0932) ccw
  line L247 (-7.7, 12.8932) -> (-7.7, 6.2932)
  arc A253 (-7, 13.5932) -> (-7.7, 12.8932) centre (-7, 12.8932) ccw
  arc A254 (-7.7, 6.2932) -> (-7, 5.5932) centre (-7, 6.2932) ccw
  arc A255 (-47.879, 1.9539) -> (-48.9397, 2.3932) centre (-48.9397, 0.8932) ccw
  arc A256 (-28.879, -0.3461) -> (-29.9397, 0.0932) centre (-29.9397, -1.4068) ccw
  arc A257 (-124.9397, 73.6932) -> (-123.879, 74.1325) centre (-124.9397, 75.1932) ccw
  arc A258 (-88.1397, 83.9932) -> (-87.079, 84.4325) centre (-88.1397, 85.4932) ccw
  arc A259 (-58.721, 83.4325) -> (-57.6603, 82.9932) centre (-57.6603, 84.4932) ccw
  arc A260 (-41.921, 81.1325) -> (-40.8603, 80.6932) centre (-40.8603, 82.1932) ccw
  line L248 (-25.7, 78.0932) -> (-25.7, 80.6932)
  line L249 (-7, 19.3955) -> (-4.4, 19.3955)
  line L250 (-111.8468, 75.9932) -> (-120.0716, 75.9932)
  line L251 (-110.4326, 76.579) -> (-104.395, 82.6166)
  arc A261 (-111.8468, 75.9932) -> (-110.4326, 76.579) centre (-111.8468, 77.9932) ccw
  arc A262 (-91.9532, 20.0932) -> (-93.3674, 19.5074) centre (-91.9532, 18.0932) ccw
  arc A263 (-74.6144, 18.5689) -> (-77.2264, 20.0932) centre (-77.2264, 17.0932) ccw
  dimension "d1" = 3.4
  dimension "d2" = 3.4
  dimension "d3" = 7.8
  dimension "d4" = 3.4
  dimension "d5" = 3.4
  dimension "d9" = 2.2
  dimension "d12" = 2.2
  dimension "d318" = 4.2
  dimension "d319" = 4.2
  constraint tangent L19 A5
  constraint tangent L19 A6
  constraint tangent L13 A7
  constraint tangent L17 A8
  constraint tangent L12 A9
  constraint tangent L16 A10
  constraint tangent L8 A11
  constraint tangent L7 A13
  constraint tangent L9 A14
  constraint tangent L18 A15
  constraint tangent L2 A16
  constraint tangent L0 A17
  constraint tangent L10 A18
  constraint tangent L5 A19
  constraint tangent L11 A20
  constraint tangent L6 A21
  constraint tangent L3 A22
  constraint tangent L1 A23
  constraint tangent L4 A24
  constraint tangent A24 L104
  constraint perpendicular L104 L105
  constraint tangent L104 A25
  constraint tangent L105 A25
  constraint coincident L15.end L105
  constraint perpendicular L15 L105
  constraint coincident L14.end L104
  constraint perpendicular L14 L104
  constraint tangent L32 A26
  constraint tangent L33 A27
  constraint tangent L35 A28
  constraint tangent L34 A29
  constraint tangent L49 A30
  constraint tangent L49 A31
  constraint tangent L51 A32
  constraint tangent L50 A33
  constraint tangent L57 A34
  constraint tangent L57 A35
  constraint tangent L59 A36
  constraint tangent L58 A37
  constraint tangent L76 A38
  constraint tangent L78 A39
  constraint tangent L79 A40
  constraint tangent L77 A41
  constraint tangent L54 A42
  constraint tangent L54 A43
  constraint tangent L52 A44
  constraint tangent L53 A45
  constraint tangent L90 A46
  constraint tangent L90 A47
  constraint tangent L91 A47
  constraint tangent L91 A48
  constraint tangent L89 A49
  constraint tangent L100 A50
  constraint tangent L101 A51
  constraint tangent L103 A52
  constraint tangent L102 A53
  constraint tangent L93 A54
  constraint tangent L93 A55
  constraint tangent L95 A56
  constraint tangent L94 A57
  constraint tangent L21 A58
  constraint tangent L20 A59
  constraint tangent L22 A59
  constraint tangent L22 A60
  constraint tangent L23 A61
  constraint tangent L64 A62
  constraint tangent L66 A62
  constraint tangent L64 A63
  constraint tangent L65 A64
  constraint tangent L67 A65
  constraint tangent L98 A66
  constraint tangent L98 A67
  constraint tangent L96 A68
  constraint tangent L97 A69
  constraint tangent L70 A70
  constraint tangent L70 A71
  constraint tangent L68 A72
  constraint tangent L69 A73
  constraint tangent L80 A74
  constraint tangent L80 A75
  constraint tangent L82 A75
  constraint tangent L82 A76
  constraint tangent L83 A76
  constraint tangent L83 A77
  constraint tangent L81 A77
  constraint tangent L29 A78
  constraint tangent L29 A79
  constraint tangent L28 A80
  constraint tangent L30 A81
  constraint tangent L37 A82
  constraint tangent L37 A83
  constraint tangent L36 A83
  constraint tangent L36 A84
  constraint tangent L38 A84
  constraint tangent L38 A85
  constraint tangent L39 A85
  constraint tangent L61 A86
  constraint tangent L61 A87
  constraint tangent L60 A87
  constraint tangent L60 A88
  constraint tangent L62 A89
  constraint tangent L40 A90
  constraint tangent L42 A91
  constraint tangent L43 A92
  constraint tangent L41 A92
  constraint tangent L41 A93
  constraint tangent L40 A93
  constraint tangent L44 A94
  constraint tangent L46 A94
  constraint tangent L46 A95
  constraint tangent L47 A95
  constraint tangent L47 A96
  constraint tangent L45 A96
  constraint tangent L45 A97
  constraint tangent L44 A97
  constraint tangent L74 A98
  constraint tangent L75 A98
  constraint tangent L74 A99
  constraint tangent L72 A100
  constraint tangent L73 A101
  constraint tangent L26 A102
  constraint tangent L27 A102
  constraint tangent L26 A103
  constraint tangent L24 A104
  constraint tangent L25 A105
  constraint tangent L86 A106
  constraint tangent L87 A106
  constraint tangent L86 A107
  constraint tangent L84 A108
  constraint tangent L85 A109
  constraint tangent A12 L107
  constraint tangent L106 A112
  constraint tangent L107 A112
  constraint concentric A8 A113
  constraint concentric A6 A114
  constraint concentric A23 A115
  constraint concentric A21 A116
  constraint parallel L108 L131
  constraint tangent A117 L131
  constraint tangent L109 A117
  constraint tangent L108 A118
  constraint tangent L109 A118
  constraint horizontal L110
  constraint perpendicular L110 L111
  constraint parallel L110 L112
  constraint parallel L111 L113
  constraint tangent A120 L113
  constraint tangent L112 A120
  constraint tangent L111 A119
  constraint tangent A119 L112
  constraint horizontal L114
  constraint perpendicular L114 L115
  constraint parallel L114 L116
  constraint parallel L115 L117
  constraint tangent A122 L117
  constraint tangent L116 A122
  constraint tangent L115 A121
  constraint tangent A121 L116
  constraint horizontal L118
  constraint perpendicular L118 L119
  constraint parallel L118 L120
  constraint parallel L119 L121
  constraint tangent A124 L121
  constraint tangent L120 A124
  constraint tangent L119 A123
  constraint tangent A123 L120
  constraint horizontal L122
  constraint perpendicular L122 L123
  constraint parallel L122 L124
  constraint parallel L123 L125
  constraint tangent A126 L125
  constraint tangent L124 A126
  constraint tangent L123 A125
  constraint tangent A125 L124
  constraint horizontal L130
  constraint perpendicular L126 L130
  constraint parallel L127 L130
  constraint parallel L126 L128
  constraint tangent A128 L128
  constraint tangent L127 A128
  constraint tangent L126 A127
  constraint tangent A127 L127
  constraint horizontal L129
  constraint perpendicular L129 L156
  constraint parallel L156 L158
  constraint tangent A132 L158
  constraint tangent A129 L129
  constraint tangent A129 L158
  constraint tangent L129 A130
  constraint tangent A130 L156
  constraint tangent A131 L156
  constraint collinear L156 L157
  constraint collinear L158 L159
  constraint tangent L157 A155
  constraint tangent L158 A156
  constraint tangent L155 A157
  constraint tangent L156 A157
  constraint tangent L155 A158
  constraint tangent L159 A158
  constraint concentric A110 A159
  constraint concentric A111 A160
  constraint tangent L15 A161
  constraint tangent L14 A161
  constraint tangent L132 A162
  constraint tangent L108 A162
  constraint tangent L131 A163
  constraint tangent L132 A163
  constraint tangent L111 A164
  constraint tangent L110 A164
  constraint tangent L113 A165
  constraint tangent L110 A165
  constraint tangent L115 A166
  constraint tangent L114 A166
  constraint tangent L117 A167
  constraint tangent L114 A167
  constraint tangent L119 A168
  constraint tangent L118 A168
  constraint tangent L121 A169
  constraint tangent L118 A169
  constraint tangent L123 A170
  constraint tangent L122 A170
  constraint tangent L125 A171
  constraint tangent L122 A171
  constraint tangent L126 A172
  constraint tangent L130 A172
  constraint tangent L130 A173
  constraint tangent L128 A173
  constraint parallel L160 L162
  constraint tangent L160 A174
  constraint tangent A174 L161
  constraint tangent A175 L162
  constraint tangent L161 A175
  constraint horizontal L164
  constraint perpendicular L164 L165
  constraint parallel L164 L166
  constraint parallel L165 L167
  constraint tangent A180 L167
  constraint tangent L166 A180
  constraint horizontal L168
  constraint perpendicular L168 L169
  constraint parallel L168 L170
  constraint parallel L169 L171
  constraint tangent A184 L171
  constraint tangent L170 A184
  constraint tangent L169 A183
  constraint tangent A183 L170
  constraint horizontal L174
  constraint perpendicular L174 L175
  constraint parallel L172 L174
  constraint parallel L173 L175
  constraint tangent A186 L173
  constraint tangent L172 A186
  constraint tangent A185 L175
  constraint tangent A185 L172
  constraint horizontal L178
  constraint perpendicular L178 L179 L39
  constraint parallel L176 L178
  constraint parallel L177 L179 L39
  constraint tangent A189 L179 L39
  constraint tangent A189 L176
  constraint horizontal L182
  constraint perpendicular L182 L183
  constraint parallel L180 L182
  constraint parallel L181 L183
  constraint tangent A193 L181
  constraint tangent L180 A193
  constraint tangent A192 L183
  constraint tangent A192 L180
  constraint tangent A176 L163
  constraint tangent L162 A176
  constraint tangent L160 A177
  constraint tangent L163 A177
  constraint tangent A179 L165
  constraint tangent L164 A179
  constraint tangent A178 L167
  constraint tangent A178 L164
  constraint tangent A182 L169
  constraint tangent L168 A182
  constraint tangent A181 L171
  constraint tangent A181 L168
  constraint tangent A188 L175
  constraint tangent L174 A188
  constraint tangent L173 A187
  constraint tangent A187 L174
  constraint tangent A191 L179 L39
  constraint tangent L178 A191
  constraint tangent L177 A190
  constraint tangent A190 L178
  constraint tangent A195 L183
  constraint tangent L182 A195
  constraint tangent A194 L182
  constraint tangent L181 A194
  constraint parallel L185 L187
  constraint tangent A199 L187
  constraint tangent L186 A199
  constraint tangent L185 A198
  constraint tangent A198 L186
  constraint horizontal L188
  constraint perpendicular L188 L189
  constraint parallel L188 L190
  constraint parallel L189 L191
  constraint tangent A202 L191
  constraint tangent L190 A202
  constraint horizontal L192
  constraint perpendicular L192 L193
  constraint parallel L192 L194
  constraint parallel L193 L195
  constraint tangent A206 L195
  constraint tangent L194 A206
  constraint tangent L193 A205
  constraint tangent A205 L194
  constraint horizontal L196
  constraint perpendicular L196 L197
  constraint parallel L196 L198
  constraint parallel L197 L199
  constraint tangent A210 L199
  constraint tangent L198 A210
  constraint tangent L197 A209 L40.start
  constraint tangent A209 L40.start L198
  constraint horizontal L200
  constraint perpendicular L200 L201
  constraint parallel L200 L202
  constraint parallel L201 L203
  constraint tangent A214 L203
  constraint tangent L202 A214
  constraint tangent L201 A213
  constraint tangent A213 L202
  constraint horizontal L204
  constraint perpendicular L204 L205
  constraint parallel L204 L206
  constraint parallel L205 L207
  constraint tangent A218 L207
  constraint tangent L206 A218
  constraint tangent L205 A217
  constraint tangent A217 L206
  constraint tangent L184 A197
  constraint tangent A197 L185
  constraint tangent A196 L187
  constraint tangent A196 L184
  constraint tangent A201 L189
  constraint tangent L188 A201
  constraint tangent A200 L191
  constraint tangent A200 L188
  constraint tangent A204 L193
  constraint tangent L192 A204
  constraint tangent A203 L195
  constraint tangent A203 L192
  constraint tangent A208 L197
  constraint tangent L196 A208
  constraint tangent A207 L199
  constraint tangent A207 L196
  constraint tangent A212 L201
  constraint tangent L200 A212
  constraint tangent A211 L203
  constraint tangent A211 L200
  constraint tangent A216 L205
  constraint tangent L204 A216
  constraint tangent A215 L204
  constraint tangent A215 L207
  constraint horizontal L209
  constraint perpendicular L208 L209
  constraint parallel L209 L218
  constraint tangent A219 L208
  constraint tangent A219 L218
  constraint horizontal L210
  constraint perpendicular L210 L213
  constraint parallel L210 L212
  constraint parallel L211 L213
  constraint tangent L211 A223
  constraint tangent A223 L212
  constraint tangent A224 L213
  constraint tangent L212 A224
  constraint tangent L208 A220
  constraint tangent A220 L209
  constraint tangent L209 A221
  constraint tangent L213 A225
  constraint tangent L210 A225
  constraint tangent L210 A222
  constraint tangent A222 L211
  constraint horizontal L214
  constraint perpendicular L214 L215
  constraint parallel L214 L216
  constraint parallel L215 L217
  constraint tangent A229 L217
  constraint tangent L216 A229
  constraint tangent L215 A228
  constraint tangent A228 L216
  constraint tangent A227 L215
  constraint tangent L214 A227
  constraint tangent A226 L214
  constraint tangent A226 L217
  constraint tangent L218 A230
  constraint tangent L220 A230
  constraint tangent L219 A231
  constraint tangent L220 A231
  constraint tangent L176 A232
  constraint tangent L221 A232
  constraint tangent L177 A233
  constraint tangent L221 A233
  constraint tangent L189 A234
  constraint tangent L222 A234
  constraint tangent L190 A235
  constraint tangent L222 A235
  constraint tangent L166 A236
  constraint tangent L223 A236
  constraint tangent L165 A237
  constraint tangent L223 A237
  constraint tangent A132 L224
  constraint tangent A156 L225
  constraint concentric A11 A238
  constraint concentric A9 A239
  constraint concentric A8 A240
  constraint concentric A6 A241
  constraint concentric A25 A242
  constraint concentric A24 A243
  constraint concentric A23 A244
  constraint concentric A21 A245
  constraint concentric A19 A246
  constraint concentric A16 A247
  constraint concentric A15 A248
  constraint concentric A14 A249
  constraint concentric A12 A250
  constraint tangent A242 L233
  constraint tangent L233 A243
  constraint tangent A238 L226
  constraint tangent A249 L241
  constraint tangent A240 L229
  constraint tangent A241 L231
  constraint tangent A248 L240
  constraint tangent A243 L234
  constraint tangent A244 L235
  constraint tangent A245 L237
  constraint tangent A247 L239
  constraint concentric A12 A133
  constraint concentric A112 A134
  constraint concentric A11 A135
  constraint concentric A10 A136
  constraint concentric A9 A137
  constraint concentric A8 A138
  constraint concentric A7 A139
  constraint concentric A6 A140
  constraint concentric A5 A141
  constraint concentric A25 A142
  constraint concentric A24 A143